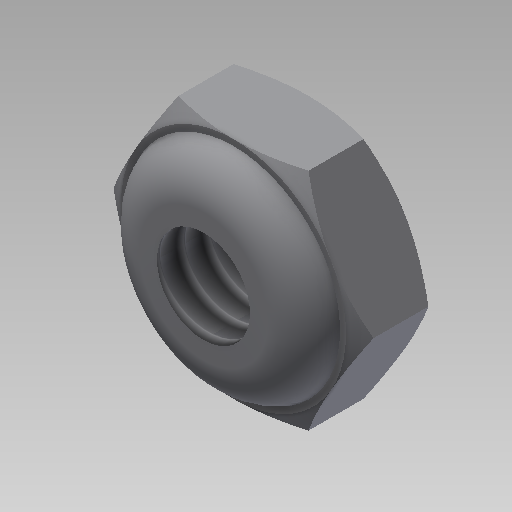
# Autodesk Inventor part: PWTR-0034
Saved by Autodesk Inventor 2020 (Build 240168000, 168)
## iProperties
Part Number: PWTR-0034
Document SubType Name: Modeling
Created: 2003-02-06
Designer: B. BOGAN
Description: LOCK NUT
Material: Default
Density: 1 g/cm^3
Mass: 0.258684 g
Surface Area: 2.9959 cm^2
Volume: 0.258684 cm^3
Appearance: Default
Vendor: Non-Design Specific
Control State: 0
Master: False
Checked Out: False
Shininess: 64.0
Length Units: 11272
Angle Units: 11279
Time Units: 11290
Mass Units: 11286
Length Display Precision: 3
Angle Display Precision: 2
Compacted: True
Density: 0.0
Volumn: 0.0
Area: 0.0
PropertySet Name: Model Information
Title: LOCK NUT
Author: B. BOGAN
Revision Number: B
Autodesk Inventor part; units mm, degrees
ref_plane "YZ Plane" through (0, 0, 0) normal (1, 0, 0) x (0, 1, 0)
ref_plane "XZ Plane" through (0, 0, 0) normal (0, 1, 0) x (-1, 0, 0)
ref_plane "XY Plane" through (0, 0, 0) normal (0, 0, 1) x (1, 0, 0)
sketch "Sketch1" plane through (0, 0, 0) normal (0, 0, 1) x (1, 0, 0)
  circle A0 centre (0, 0) radius 4.7625 construction
  line L0 (2.7496, 4.7625) -> (5.4993, 0)
  line L1 (5.4993, 0) -> (2.7496, -4.7625)
  line L2 (2.7496, -4.7625) -> (-2.7496, -4.7625)
  line L3 (-2.7496, -4.7625) -> (-5.4993, 0)
  line L4 (-5.4993, 0) -> (-2.7496, 4.7625)
  line L5 (-2.7496, 4.7625) -> (2.7496, 4.7625)
  point P0 (0, 4.7625)
  dimension "d0" = 9.525
  constraints: 12 end point, 1 coincident, 1 midpoint, 1 vertical alignment, 13 other
extrude "Extrusion1" add sketch "Sketch1" along normal blind 3.175
sketch "Sketch2" plane through (0, 0, 3.175) normal (0, 0, 1) x (1, 0, 0)
  point P0 (0, 0)
hole "Hole1" at (0, 0, 3.175) direction (0, 0, -1) diameter 3.937 end through all thread size "10-24 UNC" class "2B" standard "ANSI Unified Screw Threads"
sketch "Sketch3" plane through (0, 0, 0) normal (1, 0, 0) x (0, 1, 0)
  line L0 (-4.7625, 3.175) -> (0, 3.175) projected
  line L1 (-4.7625, 0) -> (0, 0) projected
  line L2 (-4.7625, 3.175) -> (-6.7124, 3.175)
  line L3 (-6.7124, 3.175) -> (-6.7124, 2.0492)
  line L4 (-6.7124, 2.0492) -> (-4.7625, 3.175)
  line L5 (-4.7625, 0) -> (-6.7124, 0)
  line L6 (-6.7124, 0) -> (-6.7124, 1.1258)
  line L7 (-6.7124, 1.1258) -> (-4.7625, 0)
  line L8 (0, -0.3175) -> (0, 4.1275) projected
  dimension "d10" = 30
  dimension "d11" = 30
  constraints: 12 end point, 3 perpendicular, 1 collinear, 1 parallel
  measures "d10" angle of L5 L7
  measures "d11" angle of L4 L2
revolve "Revolution1" cut sketch "Sketch3" angle 360 about axis through (0, 0, -10) along (0, 0, 1)
sketch "Sketch4" plane through (0, 0, 3.175) normal (0, 0, 1) x (1, 0, 0)
  arc A0 (4.1244, -2.3813) -> (4.1244, 2.3813) centre (0, 0) ccw projected
  arc A1 (4.1244, 2.3813) -> (0, 4.7625) centre (0, 0) ccw projected
  arc A2 (0, 4.7625) -> (-4.1244, 2.3812) centre (0, 0) ccw projected
  arc A3 (-4.1244, 2.3812) -> (-4.1244, -2.3813) centre (0, 0) ccw projected
  arc A4 (-4.1244, -2.3813) -> (0, -4.7625) centre (0, 0) ccw projected
  arc A5 (0, -4.7625) -> (4.1244, -2.3813) centre (0, 0) ccw projected
  circle A6 centre (0, 0) radius 1.9685 projected
  circle A7 centre (0, 0) radius 4.5085
  dimension "d16" = 0.254
  constraints: 1 centre point, 1 coincident, 1 concentric
  measures "d16" radial gap between concentric circles of A4 A7
extrude "Extrusion2" add sketch "Sketch4" along normal blind 1.27 contours A7
fillet "Fillet1" radius 1.905 1 edges at (-4.5085, 0, 4.445)
equation "\"d10\" = d11"
body "Solid1"
